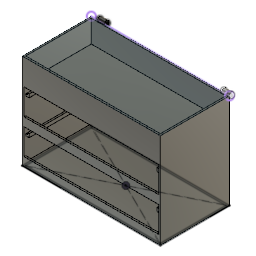
Semana4_Desafio6 (Estrutura) v1 (Autodesk Fusion 360 design; units mm, degrees)
Autodesk Fusion 360 part; units mm, degrees
sketch "Sketch1" plane through (0, 0, 0) normal (0, 0, 1) x (1, 0, 0)
  line L0 (200, -100) -> (-200, -100)
  line L1 (-200, -100) -> (-200, 100)
  line L2 (-200, 100) -> (200, 100)
  line L3 (200, 100) -> (200, -100)
  line L4 (200, -100) -> (-200, 100) construction
  line L5 (-200, -100) -> (200, 100) construction
  line L6 (195, -95) -> (-195, -95)
  line L7 (-195, -95) -> (-195, 95)
  line L8 (-195, 95) -> (195, 95)
  line L9 (195, 95) -> (195, -95)
  line L10 (195, -95) -> (-195, 95) construction
  line L11 (-195, -95) -> (195, 95) construction
  dimension "d1" = 200
  dimension "d2" = 400
  dimension "d3" = 390
  dimension "d4" = 190
  constraint horizontal L0
  constraint perpendicular L0 L1
  constraint parallel L0 L2
  constraint parallel L1 L3
  constraint coincident L4 origin
  constraint coincident L5 origin
  constraint horizontal L6
  constraint perpendicular L6 L7
  constraint parallel L6 L8
  constraint parallel L7 L9
  constraint coincident L10 origin
  constraint coincident L11 origin
  measures "d1" distance of L0.end L1.end
  measures "d2" distance of L1.end L2.end
  measures "d3" distance of L7.end L8.end
  measures "d4" distance of L6.end L7.end
extrude "Extrude1" add sketch "Sketch1" along normal blind 275
sketch "Sketch3" plane through (0, -100, 0) normal (0, -1, 0) x (1, 0, 0)
  line L0 (-200, 0) -> (200, 0)
  line L1 (200, 0) -> (200, 275)
  line L2 (200, 275) -> (-200, 275)
  line L3 (-200, 275) -> (-200, 0)
  line L4 (-195, 200) -> (195, 200)
  line L5 (195, 200) -> (195, 125)
  line L6 (195, 125) -> (-195, 125)
  line L7 (-195, 125) -> (-195, 200)
  line L8 (-195, 100) -> (195, 100)
  line L9 (195, 100) -> (195, 25)
  line L10 (195, 25) -> (-195, 25)
  line L11 (-195, 25) -> (-195, 100)
  line L12 (200, 0) -> (-200, 0)
  dimension "d11" = 5
  dimension "d12" = 5
  dimension "d13" = 25
  dimension "d14" = 25
  constraint horizontal L4
  constraint vertical L5
  constraint horizontal L6
  constraint vertical L7
  constraint horizontal L8
  constraint vertical L9
  constraint horizontal L10
  constraint vertical L11
  constraint collinear L7 L11
  constraint collinear L5 L9
  measures "d11" distance of L3 L7
  measures "d12" distance of L1 L5
  measures "d13" distance of L10 L12
  measures "d14" distance of L6 L8
extrude "Extrude2" cut sketch "Sketch3" against normal blind 10 contours L4 L5 L6 L7 | L8 L9 L10 L11
extrude "Extrude3" add sketch "Sketch1" along normal blind 10 contours L6 L7 L8 L9
ref_plane "WorkPlane1" through (0, 0, 200) normal (0, 0, 1) x (1, 0, 0)
sketch "Sketch4" plane through (0, 0, 200) normal (0, 0, 1) x (1, 0, 0)
  line L0 (200, -100) -> (-200, -100)
  line L1 (-200, -100) -> (-200, 100)
  line L2 (-200, 100) -> (200, 100)
  line L3 (200, 100) -> (200, -100)
  line L4 (200, -100) -> (-200, 100) construction
  line L5 (-200, -100) -> (200, 100) construction
  constraint horizontal L0
  constraint perpendicular L0 L1
  constraint parallel L0 L2
  constraint parallel L1 L3
  constraint coincident L4 origin
  constraint coincident L5 origin
extrude "Extrude4" add sketch "Sketch4" along normal blind 10
ref_plane "WorkPlane2" through (0, 0, 75) normal (0, 0, 1) x (1, 0, 0)
sketch "Sketch5" plane through (0, 0, 75) normal (0, 0, 1) x (1, 0, 0)
  line L0 (195, -95) -> (185, -95)
  line L1 (185, -95) -> (185, 95)
  line L2 (185, 95) -> (195, 95)
  line L3 (195, 95) -> (195, -95)
  line L4 (-195, -95) -> (-185, -95)
  line L5 (-185, -95) -> (-185, 95)
  line L6 (-185, 95) -> (-195, 95)
  line L7 (-195, 95) -> (-195, -95)
  line L8 (-190, -95) -> (-190, 95)
  line L9 (190, -95) -> (190, 95)
  line L10 (195, -95) -> (-195, -95)
  line L11 (-195, -95) -> (-195, 95)
  line L12 (-195, 95) -> (195, 95)
  line L13 (195, 95) -> (185, 95)
  line L14 (185, -95) -> (195, -95)
  dimension "d19" = 10
  dimension "d20" = 10
  dimension "d21" = 5
  dimension "d22" = 5
  constraint horizontal L0
  constraint vertical L1
  constraint horizontal L2
  constraint vertical L3
  constraint horizontal L4
  constraint vertical L5
  constraint horizontal L6
  constraint vertical L7
  constraint vertical L8
  constraint vertical L9
  constraint collinear L4 L10
  constraint coincident L8.start L10
  constraint collinear L2 L12
  constraint coincident L9.end L12
  constraint coincident L0.end L10
  constraint coincident L9.start L10
  constraint coincident L2.end L3.start
  measures "d19" distance of L0.start L0.end
  measures "d20" distance of L4.start L4.end
  measures "d21" distance of L8 L11
  measures "d22" distance of L1 L9
extrude "Extrude5" add sketch "Sketch5" along normal blind 5 contours L4 L6 L7 L8 L10 L11 L12
extrude "Extrude6" add sketch "Sketch5" along normal blind 5 contours L0 L2 L3 L9 L10 L12 L13 L14
extrude "Extrude7" add sketch "Sketch5" along normal blind 10 contours L0 L1 L2 L9 L10 L12 L13 L14 | L4 L5 L6 L8 L10 L12
ref_plane "WorkPlane3" through (0, 0, 175) normal (0, 0, 1) x (1, 0, 0)
sketch "Sketch6" plane through (0, 0, 175) normal (0, 0, 1) x (1, 0, 0)
  line L0 (-195, 95) -> (-185, 95)
  line L1 (-185, 95) -> (-185, -95)
  line L2 (-185, -95) -> (-195, -95)
  line L3 (-195, -95) -> (-195, 95)
  line L4 (-190, 95) -> (-190, -95)
  line L5 (-195, 95) -> (195, 95)
  line L6 (195, -95) -> (-195, -95)
  line L7 (195, -95) -> (185, -95)
  line L8 (185, -95) -> (185, 95)
  line L9 (185, 95) -> (195, 95)
  line L10 (195, 95) -> (195, -95)
  line L11 (190, 95) -> (190, -95)
  dimension "d30" = 5
  dimension "d31" = 5
  constraint horizontal L0
  constraint vertical L1
  constraint horizontal L2
  constraint vertical L3
  constraint vertical L4
  constraint collinear L0 L5
  constraint collinear L2 L6
  constraint coincident L4.start L5
  constraint coincident L4.end L6
  constraint midpoint L0 L4.start
  constraint horizontal L7
  constraint vertical L8
  constraint horizontal L9
  constraint vertical L10
  constraint coincident L5 L8.end
  constraint coincident L6.start L7.start
  constraint midpoint L9 L11.start
  constraint midpoint L7 L11.end
  constraint coincident L3 L0.start
  measures "d30" distance of L10 L11
  measures "d31" distance of L3 L4
extrude "Extrude8" add sketch "Sketch6" along normal blind 5 contours L0 L2 L3 L4 L5 L6 | L5 L6 L7 L9 L10 L11
extrude "Extrude9" add sketch "Sketch6" along normal blind 10 contours L0 L1 L2 L4 L5 L6 | L5 L6 L7 L8 L9 L11
sketch "Sketch7" plane through (0, 0, 275) normal (0, 0, 1) x (-1, 0, 0)
  line L0 (195, -95) -> (-195, -95)
  line L1 (-195, -95) -> (-195, 95)
  line L2 (-195, 95) -> (195, 95)
  line L3 (195, 95) -> (195, -95)
  line L4 (-200, -100) -> (200, -100)
  line L5 (200, -100) -> (200, 100)
  line L6 (200, 100) -> (-200, 100)
  line L7 (-200, 100) -> (-200, -100)
  line L8 (-179.6402, -105) -> (-199.6402, -105)
  line L9 (200, -100) -> (-200, -100)
  line L10 (180, -105) -> (160, -105)
  dimension "d36" = 5
  dimension "d37" = 5
  dimension "d50" = 20
  dimension "d51" = 20
  constraint parallel L4 L8
  constraint horizontal L10
  measures "d36" distance of L8 L9
  measures "d37" distance of L9 L10
  measures "d50" horizontal distance of L4.end L10.start
  measures "d51" distance of L10.start L10.end
pipe "Pipe2" add diameter 15 wall 2.5 path "Sketch7" along L10
pipe "Pipe3" add diameter 15 wall 2.5 path "Sketch7" along L8
